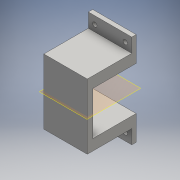
# Autodesk Inventor part: BaseClamp
Saved by Autodesk Inventor 2016 (Build 200138000, 138)
## iProperties
Created: 2017-11-27
Part Number: BaseClamp
Material: Generic
Document SubType Name: Modeling
Designer: alex
Density: 1 g/cm^3
Appearance: Default
Author: alex
Autodesk Inventor part; units mm, degrees
ref_plane "YZ Plane" through (0, 0, 0) normal (1, 0, 0) x (0, 1, 0)
ref_plane "XZ Plane" through (0, 0, 0) normal (0, 1, 0) x (-1, 0, 0)
sketch "Sketch1" plane through (0, 0, 0) normal (0, 1, 0) x (-1, 0, 0)
  line L0 (20, 30) -> (-20, 30)
  line L1 (-20, 30) -> (-20, -30)
  line L2 (-20, -30) -> (20, -30)
  line L3 (20, -30) -> (20, 30)
  point P0 (0, 0)
  point P1 (0, 30)
  point P2 (20, 0)
  dimension "d0" = 40
  dimension "d1" = 60
  constraints: 8 end point, 2 midpoint, 2 parallel, 1 horizontal, 1 horizontal alignment, 1 perpendicular, 1 vertical alignment
  measures "d0" distance of L0.start L0.end
  measures "d1" distance of L2.end L0.start
extrude "Extrusion1" add sketch "Sketch1" along normal blind 5
sketch "Sketch2" plane through (0, 5, 0) normal (0, 1, 0) x (1, 0, 0)
  line L0 (-20, -30) -> (20, -30) projected
  line L1 (20, -30) -> (20, 30) projected
  line L2 (-20, -30) -> (20, -30)
  line L3 (20, -30) -> (20, -20)
  line L4 (20, -20) -> (-20, -20)
  line L5 (-20, -20) -> (-20, -30)
  line L6 (-20, 29.9872) -> (20, 29.9872)
  line L7 (20, 29.9872) -> (20, 19.9872)
  line L8 (20, 19.9872) -> (-20, 19.9872)
  line L9 (-20, 19.9872) -> (-20, 29.9872)
  line L10 (20, 30) -> (-20, 30) projected
  point P0 (0, 0)
  dimension "d4" = 10
  dimension "d5" = 10
  dimension "d6" = 0.0128
  dimension "d7" = 40
  constraints: 16 end point, 4 parallel, 2 horizontal, 2 perpendicular, 2 point on line
  measures "d4" distance between parallel lines of L0 L4
  measures "d5" distance of L8.end L6.start
  measures "d6" distance between parallel lines of L10 L6
  measures "d7" distance between parallel lines of L9 L1
extrude "Extrusion2" add sketch "Sketch2" along normal blind 40
sketch "Sketch3" plane through (20, 5, -29.9872) normal (0, 0, -1) x (-1, 0, 0)
  line L0 (40, -5) -> (40, 40) projected
  line L1 (0, -5) -> (0, 40) projected
  line L2 (40, 40) -> (0, 40)
  line L3 (0, 40) -> (0, 36)
  line L4 (0, 36) -> (40, 36)
  line L5 (40, 36) -> (40, 40)
  point P0 (20, -5)
  dimension "d10" = 4
  constraints: 8 end point, 2 parallel, 1 horizontal, 1 perpendicular, 1 point on line
  measures "d10" distance between parallel lines of L2 L4
extrude "Extrusion3" add sketch "Sketch3" along normal blind 13
sketch "Sketch5" plane through (-20, 41, -29.9872) normal (0, -1, 0) x (1, 0, 0)
  circle A0 centre (34, -6.0128) radius 2
  circle A1 centre (6, -6.0128) radius 2
  line L0 (40, 0) -> (40, -13) projected
  line L1 (0, 0) -> (0, -13) projected
  line L2 (40, -0.0128) -> (0, -0.0128) projected
  point P0 (20, 29.9872)
  dimension "d17" = 4
  dimension "d18" = 4
  dimension "d19" = 6
  dimension "d20" = 6
  dimension "d21" = 6
  constraints: 2 centre point, 1 horizontal alignment
  measures "d17" diameter of A0
  measures "d18" diameter of A1
  measures "d19" distance from line of L0 A0.centre
  measures "d20" distance from line of L1 A1.centre
  measures "d21" distance from line of L2 A0.centre
extrude "Extrusion5" cut sketch "Sketch5" against normal through all
mirror "Mirror1" about plane through (0, 0, 0) normal (0, 0, 1) of "Extrusion3", "Extrusion5"
body "Solid1"
